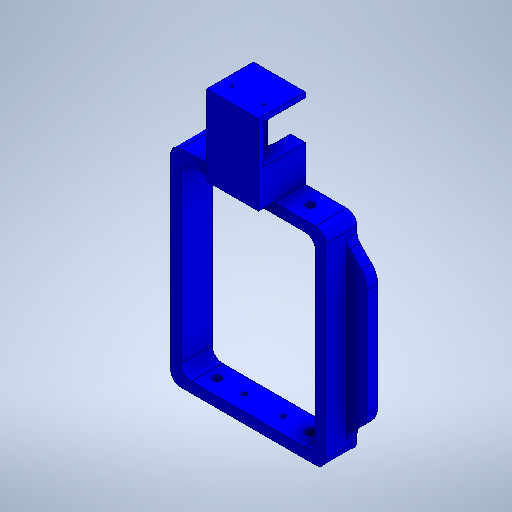
# Autodesk Inventor part: Frame
Saved by Autodesk Inventor 2025.2 (Build 292293000, 293)
## iProperties
Created: 2025-05-31
Part Number: Frame
Material: Generic
Document SubType Name: Modeling
Designer: Simon
Density: 1 g/cm^3
Appearance: Default(1)
Author: Simon
Autodesk Inventor part; units mm, degrees
ref_plane "YZ Plane" through (0, 0, 0) normal (1, 0, 0) x (0, 1, 0)
ref_plane "XZ Plane" through (0, 0, 0) normal (0, 1, 0) x (-1, 0, 0)
ref_plane "XY Plane" through (0, 0, 0) normal (0, 0, 1) x (1, 0, 0)
sketch "Sketch1" plane through (0, 0, 0) normal (0, 0, 1) x (1, 0, 0)
  line L0 (0, 0) -> (150, 0)
  line L1 (150, 0) -> (150, 200)
  line L2 (150, 200) -> (0, 200)
  line L3 (0, 200) -> (0, 0)
  line L4 (0, 0) -> (10, 0)
  line L5 (10, 0) -> (10, 10)
  line L6 (10, 10) -> (0, 10)
  line L7 (0, 10) -> (0, 0)
  line L8 (10, 10) -> (140, 10)
  line L9 (140, 10) -> (140, 190)
  line L10 (140, 190) -> (10, 190)
  line L11 (10, 190) -> (10, 10)
  line L12 (150, 200) -> (150, 160)
  line L13 (150, 160) -> (170, 160)
  line L14 (150, 0) -> (150, 40)
  line L15 (150, 40) -> (170, 40)
  line L16 (170, 40) -> (170, 160)
  line L17 (0, 200) -> (0, 160)
  line L18 (0, 160) -> (-20, 160)
  line L19 (0, 0) -> (0, 40)
  line L20 (0, 40) -> (-20, 40)
  line L21 (-20, 40) -> (-20, 160)
  line L22 (170, 160) -> (170, 180)
  line L23 (170, 180) -> (150, 180)
  line L24 (170, 160) -> (150, 180)
  line L25 (170, 40) -> (170, 20)
  line L26 (170, 20) -> (150, 20)
  line L27 (170, 40) -> (150, 20)
  line L28 (0, 40) -> (0, 20)
  line L29 (0, 20) -> (-20, 20)
  line L30 (-20, 20) -> (-20, 40)
  line L31 (-20, 40) -> (0, 20)
  line L32 (-20, 160) -> (-20, 180)
  line L33 (-20, 180) -> (0, 180)
  line L34 (0, 180) -> (-20, 160)
  point P0 (0, 180)
  dimension "d0" = 150
  dimension "d1" = 200
  dimension "d2" = 10
  dimension "d3" = 10
  dimension "d4" = 130
  dimension "d5" = 180
  dimension "d6" = 40
  dimension "d7" = 20
  dimension "d8" = 40
  dimension "d9" = 40
  dimension "d10" = 20
  dimension "d11" = 40
  constraints: 70 end point, 10 perpendicular, 7 point on line, 6 parallel, 4 midpoint, 3 horizontal, 3 vertical
  measures "d0" distance of L2.end L1.end
  measures "d1" distance of L1.end L0.end
  measures "d2" distance of L6.end L5.end
  measures "d3" distance of L5.end L4.end
  measures "d4" distance of L10.end L9.end
  measures "d5" distance of L9.end L8.end
  measures "d6" distance of L1.end L12.end
  measures "d7" distance of L12.end L13.end
  measures "d8" distance of L0.end L14.end
  measures "d9" distance of L2.end L17.end
  measures "d10" distance of L17.end L18.end
  measures "d11" distance of L0.start L19.end
extrude "Extrusion1" add sketch "Sketch1" along normal blind 30 contours L3 L6 L5 L0 | L5 L6 L3 L2 L1 L0
extrude "Extrusion2" add sketch "Sketch1" along normal blind 10 contours L31 L20 L3 | L1 L15 L27 | L20 L21 L18 L3 | L1 L13 L16 L15 | L18 L34 L3 | L1 L24 L13
fillet "Fillet1" radius 20 4 edges at (170, 160, 5) (170, 40, 5) (-20, 160, 5) (-20, 40, 5)
sketch "Sketch2" plane through (10, 10, 0) normal (0, 1, 0) x (1, 0, 0)
  line L0 (0, 0) -> (130, 0) projected
  line L1 (130, 0) -> (130, -30) projected
  line L2 (0, 0) -> (130, 0)
  line L3 (130, 0) -> (130, -30)
  line L4 (130, -30) -> (0, -30)
  line L5 (0, -30) -> (0, 0)
  line L6 (0, 0) -> (0, -30) projected
  line L7 (0, -15) -> (20, -15)
  line L8 (130, -15) -> (110, -15)
  line L9 (0, -15) -> (65, -15)
  circle A0 centre (65, -15) radius 18.65
  line L10 (46.35, -15) -> (83.65, -15)
  point P0 (-10, 0)
  dimension "d33" = 37.3
  dimension "d17" = 20
  dimension "d18" = 20
  constraints: 16 end point, 3 horizontal, 3 midpoint, 2 parallel, 2 point on line, 1 coincident, 1 horizontal alignment, 1 perpendicular, 2 other
  measures "d17" distance of L7.start L7.end
  measures "d18" distance of L8.start L8.end
hole "Hole1" at (30, 10, 15) at (120, 10, 15) direction (0, -1, 0) diameter 8 depth 5
hole "Hole2" at (120, 10, 15) at (30, 10, 15) direction (0, 1, 0) diameter 8 end through all
hole "Hole3" at (56.35, 10, 15) at (93.65, 10, 15) direction (0, -1, 0) diameter 5 end through all
hole "Hole4" at (75, 10, 15) direction (0, 1, 0) diameter 22 end through all
sketch "Sketch3" plane through (0, 200, 0) normal (0, 1, 0) x (1, 0, 0)
  point P0 (0, 0)
sketch "Sketch4" plane through (0, 200, 0) normal (0, 1, 0) x (1, 0, 0)
  point P0 (0, 0)
sketch "Sketch5" plane through (0, 200, 0) normal (0, 1, 0) x (1, 0, 0)
  line L0 (150, 0) -> (0, 0) projected
  line L1 (60, -30.0202) -> (90, -30.0202)
  line L2 (90, -30.0202) -> (90, 0)
  line L3 (90, 0) -> (60, 0)
  line L4 (60, 0) -> (60, -30.0202)
  line L5 (60, -30.0202) -> (90, 0) construction
  line L6 (90, -30.0202) -> (60, 0) construction
  line L7 (60, -30.0202) -> (90, -30.0202)
  line L8 (90, -30.0202) -> (90, -45.0202)
  line L9 (90, -45.0202) -> (60, -45.0202)
  line L10 (60, -45.0202) -> (60, -30.0202)
  circle A0 centre (75, -15.0101) radius 11
  line L11 (50, -30.0202) -> (100, -30.0202)
  line L12 (100, -30.0202) -> (100, 0)
  line L13 (100, 0) -> (50, 0)
  line L14 (50, 0) -> (50, -30.0202)
  line L15 (50, -30.0202) -> (100, 0) construction
  line L16 (100, -30.0202) -> (50, 0) construction
  line L17 (50, -30.0202) -> (100, -30.0202)
  line L18 (100, -30.0202) -> (100, -45.0202)
  line L19 (100, -45.0202) -> (50, -45.0202)
  line L20 (50, -45.0202) -> (50, -30.0202)
  line L21 (86, -15.0101) -> (86, 0)
  line L22 (64, -15.0101) -> (64, 0)
  line L23 (64, 0) -> (64, 0.05)
  line L24 (64, 0.05) -> (86, 0.05)
  line L25 (86, 0.05) -> (86, 0)
  point P0 (90, -45.0202)
  point P1 (60, -45.0202)
  point P2 (86, 0)
  point P3 (64, 0)
  dimension "d48" = 30
  dimension "d49" = 15
  dimension "d52" = 50
  dimension "d53" = 15
  dimension "d54" = 50
  dimension "d72" = 0.05
  constraints: 50 end point, 9 parallel, 7 perpendicular, 6 point on line, 4 horizontal, 4 midpoint, 2 point on circle, 1 centre point, 1 coincident
  measures "d48" distance of L3.end L2.end
  measures "d49" distance of L7.end L8.end
  measures "d52" distance of L13.end L12.end
  measures "d53" distance of L17.end L18.end
  measures "d54" distance of L18.end L19.end
  measures "d72" distance of L22.end L23.end
extrude "Extrusion3" add sketch "Sketch5" along normal blind 35 contours L12 L11 L2 L0 | L2 L1 L4 L0 L22 A0 L21 | L18 L19 L8 L11 | L8 L9 L10 L1 | L11 L14 L0 L4 | L10 L19 L20 L11
sketch "Sketch6" plane through (0, 235, 0) normal (0, 1, 0) x (1, 0, 0)
  line L0 (50, -45.0202) -> (100, -45.0202) projected
  line L1 (50, 0) -> (50, -45.0202) projected
  line L2 (100, -45.0202) -> (50, -45.0202)
  line L3 (50, -45.0202) -> (50, -40.0202)
  line L4 (50, -40.0202) -> (100, -40.0202)
  line L5 (100, -40.0202) -> (100, -45.0202)
  line L6 (50, -15) -> (100, -15)
  circle A0 centre (75, -15) radius 11
  arc A1 (86, -15.0101) -> (64, -15) centre (75, -15) ccw projected
  line L7 (64, -15) -> (64, 0)
  line L8 (64, 0) -> (86, -15.0101)
  line L9 (86, -15.0101) -> (86, 0)
  circle A2 centre (75, -15) radius 21.75
  line L10 (75, -15) -> (90.3796, -30.3796)
  line L11 (75, -15) -> (96.75, -15) construction
  line L12 (75, -15) -> (59.6204, -30.3796)
  line L13 (86, 0) -> (64, 0)
  line L14 (10, 0) -> (140, 0) projected
  point P0 (0, 0)
  dimension "d55" = 5
  dimension "d56" = 43.5
  dimension "d57" = 45
  constraints: 24 end point, 3 horizontal, 3 parallel, 2 coincident, 2 point on circle, 1 centre point, 1 collinear, 1 equal length, 1 midpoint, 1 perpendicular, 1 point on line, 1 tangent, 1 vertical, 2 other
  measures "d55" distance of L2.end L3.end
  measures "d56" diameter of A2
  measures "d57" angle of L10 L11
extrude "Extrusion4" add sketch "Sketch6" along normal blind 37.3 contours L1 L4 L5 L0
sketch "Sketch7" plane through (0, 272.3, 0) normal (0, 1, 0) x (1, 0, 0)
  line L0 (50, -30) -> (50, -45.0202) projected
  line L1 (140, 0) -> (10, 0) projected
  line L2 (50, -45.0202) -> (100, -45.0202)
  line L3 (100, -45.0202) -> (100, 0)
  line L4 (100, 0) -> (50, 0)
  line L5 (50, 0) -> (50, -45.0202)
  point P0 (0, 0)
  dimension "d60" = 50
  constraints: 8 end point, 2 parallel, 1 horizontal, 1 perpendicular, 1 point on line
  measures "d60" distance of L4.end L3.end
extrude "Extrusion5" add sketch "Sketch7" along normal blind 5
hole "Hole5" at (90.3796, 235, 30.3796) at (59.6204, 235, 30.3796) direction (0, 1, 0) diameter 3 end through all
fillet "Fillet2" radius 10 4 edges at (150, 180, 5) (150, 20, 5) (0, 20, 5) (0, 180, 5)
fillet "Fillet3" radius 10 8 edges at (150, 200, 15) (150, 0, 15) (140, 10, 15) (0, 0, 15) (0, 200, 15) (140, 190, 15) (10, 10, 15) (10, 190, 15)
sketch "Sketch8" plane through (64, 200, 0) normal (0, 1, 0) x (1, 0, 0)
  circle A0 centre (11, -15) radius 11 projected
  circle A1 centre (11, -15) radius 11
  line L0 (22, -15.0101) -> (22, 0) projected
  line L1 (11, -15) -> (22, -15)
  line L2 (22, -15) -> (22, 0)
  line L3 (22, 0) -> (11, 0)
  line L4 (11, 0) -> (11, -15)
  line L5 (11, -15) -> (0, -15)
  line L6 (0, -15) -> (0, 0)
  line L7 (0, 0) -> (11, 0)
  line L8 (11, 0) -> (11, -15)
  point P0 (-64, 0)
  constraints: 16 end point, 4 parallel, 2 horizontal, 2 perpendicular, 1 centre point, 1 coincident, 1 point on line, 1 other
extrude "Extrusion6" cut sketch "Sketch8" against normal blind 50 contours L6 L7 L4 A0 | A0 L4 L5 | L4 L3 L0 A0 | A0 L1 L4
body "Solid1"
